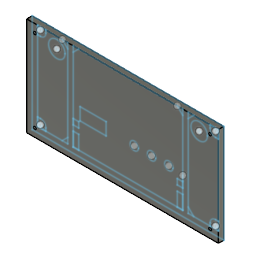
RP-couvercle-v1 (Autodesk Fusion 360 design; units mm, degrees)
part number: 2026-01-11-12-27-13-047
Autodesk Fusion 360 part; units mm, degrees
sketch "Esquisse1" plane through (0, 0, 0) normal (0, 1, 0) x (1, 0, 0)
  line L0 (-35, 18) -> (35, 18)
  line L1 (35, 18) -> (35, -18)
  line L2 (35, -18) -> (-35, -18)
  line L3 (-35, -18) -> (-35, 18)
  line L4 (-33, -16) -> (-22, -16)
  line L5 (-22, -16) -> (-22, 16)
  line L6 (-22, 16) -> (-33, 16)
  line L7 (-33, 16) -> (-33, -16)
  line L8 (33, -16) -> (22, -16)
  line L9 (22, -16) -> (22, 16)
  line L10 (22, 16) -> (33, 16)
  line L11 (33, 16) -> (33, -16)
  line L12 (-20, -16) -> (20, -16)
  line L13 (20, -16) -> (20, 16)
  line L14 (20, 16) -> (-20, 16)
  line L15 (-20, 16) -> (-20, -16)
  line L16 (32, -13) -> (33, -13)
  line L17 (33, -13) -> (33, -16)
  line L18 (33, -16) -> (30, -16)
  line L19 (30, -16) -> (30, -15)
  line L20 (32, 13) -> (33, 13)
  line L21 (33, 13) -> (33, 16)
  line L22 (33, 16) -> (30, 16)
  line L23 (30, 16) -> (30, 15)
  circle A0 centre (26, -12) radius 3
  arc A1 (32, -13) -> (30, -15) centre (32, -15) ccw
  arc A2 (30, 15) -> (32, 13) centre (32, 15) ccw
  line L24 (24, -16) -> (22, -14)
  line L25 (22, 14) -> (24, 16)
  line L26 (18, -16) -> (20, -14)
  line L27 (-18, -16) -> (-20, -14)
  line L28 (-22, 14) -> (-24, 16)
  line L29 (-24, -16) -> (-22, -14)
  line L30 (-33, -16) -> (-30, -16)
  line L31 (-30, -16) -> (-30, -15)
  line L32 (-32, -13) -> (-33, -13)
  line L33 (-33, -13) -> (-33, -16)
  line L34 (-32, 13) -> (-33, 13)
  line L35 (-33, 13) -> (-33, 16)
  line L36 (-33, 16) -> (-30, 16)
  line L37 (-30, 16) -> (-30, 15)
  arc A3 (-30, -15) -> (-32, -13) centre (-32, -15) ccw
  arc A4 (-32, 13) -> (-30, 15) centre (-32, 15) ccw
  circle A5 centre (-26, -12) radius 3
  line L38 (-20, 16) -> (-18, 16)
  line L39 (-18, 16) -> (-18, 11)
  line L40 (-18, 11) -> (-20, 11)
  line L41 (-20, 11) -> (-20, 16)
  line L42 (18, 11) -> (20, 11)
  line L43 (20, 11) -> (20, 16)
  line L44 (20, 16) -> (18, 16)
  line L45 (18, 16) -> (18, 11)
  line L46 (20, 9) -> (18, 9)
  line L47 (18, 9) -> (18, 7)
  line L48 (18, 7) -> (20, 7)
  line L49 (20, 7) -> (20, 9)
  line L50 (-18, 9) -> (-20, 9)
  line L51 (-20, 9) -> (-20, 7)
  line L52 (-20, 7) -> (-18, 7)
  line L53 (-18, 7) -> (-18, 9)
  line L54 (-17.5, 6.5) -> (-8, 6.5)
  line L55 (-8, 6.5) -> (-8, 2)
  line L56 (-8, 2) -> (-17.5, 2)
  line L57 (-17.5, 2) -> (-17.5, 6.5)
  line L58 (20, 5) -> (20, 6.5)
  circle A6 centre (14.9, 4.5) radius 1.5
  circle A7 centre (8.6, 4.5) radius 1.5
  circle A8 centre (2.3, 4.5) radius 1.5
  circle A9 centre (-32, -15) radius 0.5
  circle A10 centre (-32, 15) radius 0.5
  circle A11 centre (32, -15) radius 0.5
  circle A12 centre (32, 15) radius 0.5
  circle A13 centre (-26, -12) radius 0.5
  circle A14 centre (26, -12) radius 0.5
  constraint coincident L8 L24.start
  constraint coincident L9 L24.end
  constraint coincident L9 L25.start
  constraint coincident L10 L25.end
  constraint coincident L13 L26.end
  constraint coincident L12 L27.start
  constraint coincident L15 L27.end
  constraint coincident L5 L28.start
  constraint coincident L6 L28.end
  constraint coincident L5 L29.end
  constraint coincident L13 L46.start
  constraint coincident L15 L51.end
  constraint coincident L13 L58.end
extrude "Extrusion8" add sketch "Esquisse1" along normal blind 2 contours L4 L5 L6 L7 L28 L29 L31 L32 L34 L37 A3 A4 | L8 L9 L10 L11 L16 L19 L20 L23 A1 A2 L24 L25 | L12 L13 L14 L15 L26 L27 L39 L40 L42 L45 L46 L47 L48 L50 L52 L53 L58 | A0 | A5 | L54 L55 L56 L57 | A6 | A7 | A8 | A13 | A14 makes body 1 at (-25.0564, 0, 4.3936) makes body 2 at (-6, 0, 8.3333) makes body 3 at (25.0564, 0, -4.3936)
extrude "Extrusion9" add sketch "Esquisse1" against normal blind 2 separate body contours L0 L1 L2 L3 | L4 L7 L30 L31 L32 L33 A3 | L4 L5 L6 L7 L28 L29 L31 L32 L34 L37 A3 A4 | L4 L5 L29 | L6 L7 L34 L35 L36 L37 A4 | L5 L6 L28 | L8 L11 L16 L17 L18 L19 A1 | L8 L9 L10 L11 L16 L19 L20 L23 A1 A2 L24 L25 | L8 L9 L24 | L10 L11 L20 L21 L22 L23 A2 | L9 L10 L25 | L12 L15 L27 | L12 L13 L14 L15 L26 L27 L39 L40 L42 L45 L46 L47 L48 L50 L52 L53 L58 | L12 L13 L26 | L15 L50 L51 L52 L53 | L14 L15 L38 L39 L40 L41 | L13 L46 L47 L48 L49 | L13 L14 L42 L43 L44 L45 | A0 | A5 | L54 L55 L56 L57 | A6 | A7 | A8 | A13 | A14 makes body 4
